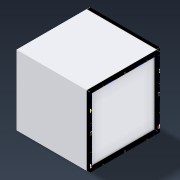
# Autodesk Inventor part: куб для форжа
Saved by Autodesk Inventor 2021 (Build 250183000, 183)
## iProperties
Created: 2020-11-11
Part Number: куб для форжа
Material: Типовые
Document SubType Name: Modeling
Designer: Daniel
Density: 1 g/cm^3
Appearance: По умолчанию
Author: Daniel
Autodesk Inventor part; units mm, degrees
ref_plane "YZ Plane" through (0, 0, 0) normal (1, 0, 0) x (0, 1, 0)
ref_plane "XZ Plane" through (0, 0, 0) normal (0, 1, 0) x (-1, 0, 0)
sketch "Эскиз1" plane through (0, 0, 0) normal (0, 1, 0) x (-1, 0, 0)
  line L0 (0, 0) -> (100, 0)
  line L1 (100, 0) -> (100, -100)
  line L2 (100, -100) -> (0, -100)
  line L3 (0, -100) -> (0, 0)
  dimension "d0" = 100
  dimension "d1" = 100
  constraints: 8 end point, 2 parallel, 1 horizontal, 1 perpendicular
  measures "d0" distance of L1.end L2.end
  measures "d1" distance of L0.end L1.end
extrude "Выдавливание1" add sketch "Эскиз1" along normal blind 100
sketch "Эскиз2" plane through (0, 0, 0) normal (1, 0, 0) x (0, 0, -1)
  line L0 (0, 0) -> (100, 0) projected
  line L1 (100, 0) -> (100, 100) projected
  line L2 (0, 100) -> (100, 100) projected
  line L3 (0, 0) -> (0, 100) projected
  line L4 (97, 97) -> (97, 3)
  line L5 (97, 3) -> (3, 3)
  line L6 (3, 3) -> (3, 97)
  line L7 (3, 97) -> (97, 97)
  dimension "d4" = 3
  constraints: 8 end point, 3 other
  measures "d4" distance between parallel lines of L2 L7
extrude "Выдавливание2" add sketch "Эскиз2" along normal blind 5 separate body
sketch "Эскиз3" plane through (0, 0, -100) normal (0, 0, -1) x (-1, 0, 0)
  line L0 (-25.4002, 113.6214) -> (124.5998, 113.6214) construction
  line L1 (124.5998, 113.6214) -> (124.5998, -8.2826) construction
  line L2 (124.5998, -8.2826) -> (-25.4002, -8.2826) construction
  line L3 (-25.4002, -8.2826) -> (-25.4002, 113.6214) construction
  line L4 (0, 100) -> (100, 100) projected
  line L5 (50, 100) -> (50, 0) construction
  line L6 (0, 0) -> (100, 0) projected
  line L7 (50, 85.9269) -> (51.8817, 85.9269)
  line L8 (51.8817, 85.9269) -> (51.8817, 99.1464)
  line L9 (51.8817, 99.1464) -> (99.4238, 99.1464)
  line L10 (99.4238, 99.1464) -> (99.4238, 69.5479)
  line L11 (99.4238, 69.5479) -> (81.1226, 69.5479)
  line L12 (81.1226, 69.5479) -> (81.1226, 56.9147)
  line L13 (81.1226, 56.9147) -> (100, 56.9147)
  line L14 (100, 0) -> (100, 100) projected
  line L15 (100, 57.8646) -> (82.0334, 57.8646)
  line L16 (82.0334, 57.8646) -> (82.0334, 68.6776)
  line L17 (82.0334, 68.6776) -> (100, 68.4983)
  line L18 (100, 68.4983) -> (100, 100)
  line L19 (100, 100) -> (50, 100)
  line L20 (59.3518, 91.7709) -> (73.7746, 91.7709)
  line L21 (73.7746, 91.7709) -> (73.7746, 86.6905)
  line L22 (73.7746, 86.6905) -> (59.3518, 86.6905)
  line L23 (59.3518, 86.6905) -> (59.3518, 91.7709)
  line L24 (81.6509, 91.7709) -> (92.3572, 91.7709)
  line L25 (92.3572, 91.7709) -> (92.3572, 86.6905)
  line L26 (92.3572, 86.6905) -> (81.6509, 86.6905)
  line L27 (81.6509, 86.6905) -> (81.6509, 91.7709)
  line L28 (74.5247, 92.521) -> (58.6016, 92.521)
  line L29 (58.6016, 92.521) -> (58.6016, 85.9404)
  line L30 (58.6016, 85.9404) -> (74.5247, 85.9404)
  line L31 (74.5247, 85.9404) -> (74.5247, 92.521)
  line L32 (93.1755, 92.5892) -> (80.8326, 92.5892)
  line L33 (80.8326, 92.5892) -> (80.8326, 85.8722)
  line L34 (80.8326, 85.8722) -> (93.1755, 85.8722)
  line L35 (93.1755, 85.8722) -> (93.1755, 92.5892)
  line L36 (81.6509, 76.917) -> (92.3572, 76.917)
  line L37 (92.3572, 76.917) -> (92.3572, 78.8687)
  line L38 (92.3572, 78.8687) -> (81.6509, 78.8687)
  line L39 (81.6509, 78.8687) -> (81.6509, 76.917)
  line L40 (80.9495, 79.5701) -> (93.0586, 79.5701)
  line L41 (93.0586, 79.5701) -> (93.0586, 76.2156)
  line L42 (93.0586, 76.2156) -> (80.9495, 76.2156)
  line L43 (80.9495, 76.2156) -> (80.9495, 79.5701)
  line L44 (70.5075, 37.9508) -> (73.7746, 37.9508)
  line L45 (73.7746, 37.9508) -> (73.7746, 49.5787)
  line L46 (73.7746, 49.5787) -> (70.5075, 49.5787)
  line L47 (70.5075, 49.5787) -> (70.5075, 37.9508)
  line L48 (74.4665, 50.2706) -> (74.4665, 37.2589)
  line L49 (74.4665, 37.2589) -> (69.8156, 37.2589)
  line L50 (69.8156, 37.2589) -> (69.8156, 50.2706)
  line L51 (69.8156, 50.2706) -> (74.4665, 50.2706)
  line L52 (59.3518, 28.1457) -> (73.7746, 28.1457)
  line L53 (73.7746, 28.1457) -> (73.7746, 30.0465)
  line L54 (73.7746, 30.0465) -> (59.3518, 30.0465)
  line L55 (59.3518, 30.0465) -> (59.3518, 28.1457)
  line L56 (58.6503, 30.7479) -> (74.4761, 30.7479)
  line L57 (74.4761, 30.7479) -> (74.4761, 27.4443)
  line L58 (74.4761, 27.4443) -> (58.6503, 27.4443)
  line L59 (58.6503, 27.4443) -> (58.6503, 30.7479)
  line L60 (70.5075, 78.7866) -> (73.7746, 78.7866)
  line L61 (73.7746, 78.7866) -> (73.7746, 57.3903)
  line L62 (73.7746, 57.3903) -> (70.5075, 57.3903)
  line L63 (70.5075, 57.3903) -> (70.5075, 78.7866)
  line L64 (70.5075, 68.9995) -> (70.5075, 67.18)
  line L65 (69.8229, 79.4713) -> (74.4593, 79.4713)
  line L66 (74.4593, 79.4713) -> (74.4593, 56.7056)
  line L67 (74.4593, 56.7056) -> (69.8229, 56.7056)
  line L68 (69.8229, 69.7638) -> (58.5875, 69.7638)
  line L69 (58.5875, 69.7638) -> (58.5875, 66.4157)
  line L70 (58.5875, 66.4157) -> (69.8229, 66.4157)
  line L71 (69.8229, 56.7056) -> (69.8229, 66.4157)
  line L72 (69.8229, 69.7638) -> (69.8229, 79.4713)
  line L73 (85.6323, 30.7509) -> (80.9465, 30.7509)
  line L74 (80.9465, 30.7509) -> (80.9465, 17.683)
  line L75 (80.9465, 17.683) -> (85.8008, 17.683)
  line L76 (85.6323, 30.7479) -> (93.0852, 30.7479)
  line L77 (93.0852, 30.7479) -> (93.0641, 27.3826)
  line L78 (93.0641, 27.3826) -> (85.8008, 27.3826)
  line L79 (85.8008, 17.683) -> (85.8008, 27.3826)
  line L80 (85.6323, 30.7479) -> (85.6323, 30.7509)
  line L81 (74.4593, 21.0609) -> (69.7036, 21.0609)
  line L82 (69.7036, 21.0609) -> (69.7036, 11.2314)
  line L83 (69.7036, 11.2314) -> (58.5875, 11.2314)
  line L84 (58.5875, 11.2314) -> (58.5875, 7.8306)
  line L85 (58.5875, 7.8306) -> (93.0852, 7.8306)
  line L86 (93.0852, 7.8306) -> (93.0852, 11.2314)
  line L87 (93.0852, 11.2314) -> (74.4593, 11.2314)
  line L88 (74.4593, 11.2314) -> (74.4593, 21.0609)
  line L89 (92.0037, 21.0609) -> (92.0037, 17.683)
  line L90 (92.0037, 17.683) -> (99.4238, 17.683)
  line L91 (99.4238, 17.683) -> (99.4238, 1.5858)
  line L92 (99.4238, 1.5858) -> (50, 1.5858)
  line L93 (92.0037, 21.0609) -> (99.4238, 21.0609)
  line L94 (99.4238, 21.0609) -> (99.4238, 37.2589)
  line L95 (99.4238, 37.2589) -> (80.9465, 37.2589)
  line L96 (80.9465, 37.2589) -> (80.9465, 50.2706)
  line L97 (80.9465, 50.2706) -> (100, 50.2706)
  line L98 (100, 56.9147) -> (100, 57.8646)
  line L99 (50, 1.5858) -> (50, 0)
  line L100 (50, 0) -> (100, 0)
  line L101 (100, 0) -> (100, 50)
  line L102 (50, 85.9269) -> (50, 100)
  line L103 (53.1286, 59.9424) -> (63.2809, 59.9424)
  line L104 (63.2809, 59.9424) -> (63.2809, 46.9528)
  line L105 (63.2809, 46.9528) -> (50, 46.9528)
  line L106 (50, 46.9528) -> (50, 48.386)
  line L107 (50, 48.386) -> (61.9322, 48.386)
  line L108 (61.9322, 48.386) -> (61.9322, 58.6353)
  line L109 (61.9322, 58.6353) -> (53.1286, 58.6353)
  line L110 (53.1286, 58.6353) -> (53.1286, 59.9424)
  line L111 (50, 79.5701) -> (63.2809, 79.5701)
  line L112 (63.2809, 79.5701) -> (63.2809, 76.0454)
  line L113 (63.2809, 76.0454) -> (52.1933, 76.2156)
  line L114 (52.1933, 76.2156) -> (52.1933, 66.4157)
  line L115 (52.1933, 66.4157) -> (50, 66.4157)
  line L116 (50, 66.4157) -> (50, 79.5701)
  line L117 (50, 7.8306) -> (52.1933, 7.8306)
  line L118 (52.1933, 7.8306) -> (52.1933, 17.683)
  line L119 (52.1933, 17.683) -> (63.2809, 17.683)
  line L120 (63.2809, 17.683) -> (63.2809, 21.0609)
  line L121 (63.2809, 21.0609) -> (50, 21.0609)
  line L122 (50, 7.8306) -> (50, 21.0609)
  line L123 (50, 40.547) -> (63.2809, 40.547)
  line L124 (63.2809, 40.547) -> (63.2809, 37.2589)
  line L125 (63.2809, 37.2589) -> (52.1933, 37.2589)
  line L126 (52.1933, 37.2589) -> (52.1933, 27.3826)
  line L127 (52.1933, 27.3826) -> (50, 27.3826)
  line L128 (50, 27.3826) -> (50, 40.547)
  dimension "d12" = 150
  dimension "d16" = 121.904
  constraints: 242 end point, 42 perpendicular, 32 parallel, 24 point on line, 15 horizontal, 5 vertical, 4 collinear, 3 midpoint, 32 other
  measures "d12" distance of L0.start L0.end
  measures "d16" distance of L0.end L1.end
extrude "Выдавливание3" add sketch "Эскиз3" along normal blind 5 separate body contours L14 L6 L99 L92 L91 L90 L89 L93 L94 L95 L96 L97 | L4 L14 L17 L16 L15 L13 L12 L11 L10 L9 L8 L7 L102 | L14 L15 L16 L17 | L20 L21 L22 L23 | L24 L25 L26 L27 | L31 L30 L29 L28 | L35 L34 L33 L32 | L39 L38 L37 L36 | L40 L41 L42 L43 | L47 L46 L45 L44 | L48 L49 L50 L51 | L55 L54 L53 L52 | L56 L57 L58 L59 | L60 L61 L62 L63 | L65 L66 L67 L71 L70 L69 L68 L72 | L80 L76 L77 L78 L79 L75 L74 L73 | L88 L87 L86 L85 L84 L83 L82 L81 | L103 L104 L105 L106 L107 L108 L109 L110 | L111 L112 L113 L114 L115 L116 | L122 L121 L120 L119 L118 L117 | L123 L124 L125 L126 L127 L128
ref_plane "РабПлоскость1" through (-50, 0, -100) normal (-1, 0, 0) x (0, 0, 1)
mirror "Зеркальное отражение1" about plane through (-50, 0, -100) normal (-1, 0, 0) of "Выдавливание3" bodies 3
